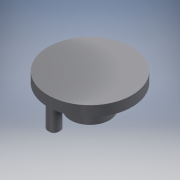
# Autodesk Inventor part: Cup_Dispenser_Transmission
Saved by Autodesk Inventor 2016 (Build 200138000, 138)
## iProperties
Created: 2015-07-04
Part Number: Cup_Dispenser_Transmission
Material: Generic
Document SubType Name: Modeling
Designer: marku
Density: 1 g/cm^3
Appearance: Default
Author: marku
Autodesk Inventor part; units mm, degrees
ref_plane "YZ Plane" through (0, 0, 0) normal (1, 0, 0) x (0, 1, 0)
ref_plane "XY Plane" through (0, 0, 0) normal (0, 0, 1) x (1, 0, 0)
ref_plane "Work Plane1" through (0, 0, 0) normal (0, 0, 1) x (1, 0, 0)
sketch "Sketch1" plane through (0, 0, 0) normal (0, 0, 1) x (1, 0, 0)
  circle A0 centre (0, -82) radius 9.5
  circle A1 centre (0, -99.5) radius 3
  circle A2 centre (0, -82) radius 2.5 projected
  line L0 (-8.4261, -52.5) -> (8.4261, -52.5) projected
  arc A3 (8.4261, -52.5) -> (35, -25.9261) centre (0, -17.5) ccw projected
  line L1 (35, -25.9261) -> (35, 1.9884) projected
  line L2 (35, 1.9884) -> (31.375, 1.9884) projected
  line L3 (31.375, 1.9884) -> (31.375, 17.5) projected
  arc A4 (31.375, 17.5) -> (-31.375, 17.5) centre (0, 17.5) ccw projected
  line L4 (-31.375, 17.5) -> (-31.375, 1.9884) projected
  line L5 (-31.375, 1.9884) -> (-35, 1.9884) projected
  line L6 (-35, 1.9884) -> (-35, -25.9261) projected
  arc A5 (-35, -25.9261) -> (-8.4261, -52.5) centre (0, -17.5) ccw projected
  arc A6 (16, -105.5) -> (36, -85.5) centre (16, -85.5) ccw projected
  line L7 (-16, -105.5) -> (16, -105.5) projected
  arc A7 (-36, -85.5) -> (-16, -105.5) centre (-16, -85.5) ccw projected
  line L8 (-36, -55.5) -> (-36, -85.5) projected
  line L9 (-38, -53.5) -> (-36, -55.5) projected
  line L10 (-38, -53.5) -> (-38, 58.5) projected
  line L11 (38, 58.5) -> (-38, 58.5) projected
  line L12 (38, -53.5) -> (38, 58.5) projected
  line L13 (36, -55.5) -> (38, -53.5) projected
  line L14 (36, -55.5) -> (36, -85.5) projected
  arc A8 (17.5, -102.5) -> (17.5, -96.5) centre (17.5, -99.5) ccw projected
  line L15 (17.5, -96.5) -> (-17.5, -96.5) projected
  arc A9 (-17.5, -96.5) -> (-17.5, -102.5) centre (-17.5, -99.5) ccw projected
  line L16 (-17.5, -102.5) -> (17.5, -102.5) projected
  line L17 (-20.5, -99.5) -> (20.5, -99.5) construction
  line L18 (0, -96.5) -> (0, -102.5) construction
  circle A10 centre (20.939, -64.9505) radius 8.4511 projected
  circle A11 centre (-20.939, -64.9505) radius 8.4511 projected
  circle A12 centre (0, -82) radius 11.5 projected
  point P0 (0, 0)
  dimension "d5" = 6
  constraints: 4 end point, 3 midpoint, 2 centre point, 2 point on circle, 1 coincident
  measures "d5" diameter of A1
extrude "Extrusion1" add sketch "Sketch1" against normal blind 10 contours A0 | A1
sketch "Sketch2" plane through (0, -82, 0) normal (0, 0, 1) x (1, 0, 0)
  circle A0 centre (0, 0) radius 20.5
  circle A1 centre (0, 0) radius 2.5 projected
  point P0 (0, 82)
  dimension "d22" = 41
  constraints: 1 centre point, 1 coincident
  measures "d22" diameter of A0
extrude "Extrusion2" add sketch "Sketch2" along normal blind 3
chamfer "Chamfer1" distance 1 angle 45 1 edges at (-3, -99.5, -10)
sketch "Sketch3" plane through (0, -82, 3) normal (0, 0, 1) x (1, 0, 0)
  circle A0 centre (0, 0) radius 20.5 projected
  circle A1 centre (0, 0) radius 2.5 projected
  point P0 (0, 82)
ref_plane "Work Plane2" through (-3.7976, -85.7976, 4.5) normal (0, 0, 1) x (1, 0, 0)
ref_plane "Work Plane3" through (-116.9481, -147.3506, 6) normal (0, 0, 1) x (1, 0, 0)
extrude "Extrusion3" add sketch "Sketch3" along normal up to surface (3 mm away) contours A0 | A1
thicken "Thicken1" operation add thickness 0.1 both sides no extend neighbours yes toward (0.1226408, 0.9924511, 0) faces at (-0.3679, -102.4774, -3) (-2.5141, -102.3452, 2)
thicken "Thicken2" operation add thickness 1 both sides no extend neighbours yes toward (0, 0, 1) faces at (6.049, -95.8683, 0)
ref_plane "Work Plane4" through (0, -72.5, 0) normal (0, 1, 0) x (-1, 0, 0)
sketch "Sketch5" plane through (0, -72.5, 0) normal (0, 1, 0) x (-1, 0, 0)
  circle A0 centre (0, -5) radius 1.5
  point P0 (0, 0)
  dimension "d19" = 3
  constraints: 1 centre point
  measures "d19" diameter of A0
extrude "Extrusion5" cut sketch "Sketch5" against normal up to next
body "Solid1"
